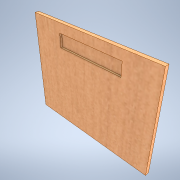
# Autodesk Inventor part: DoosjeVoorkant
Saved by Autodesk Inventor 2021 (Build 250183000, 183)
## iProperties
Created: 2021-03-11
Part Number: DoosjeVoorkant
Material: Wood (Cherry)
Document SubType Name: Modeling
Designer: ZiweZhang
Density: 0.63 g/cm^3
Appearance: Cherry - Natural Low Gloss
Author: ZiweZhang
Autodesk Inventor part; units mm, degrees
ref_plane "YZ Plane" through (0, 0, 0) normal (1, 0, 0) x (0, 1, 0)
ref_plane "XZ Plane" through (0, 0, 0) normal (0, 1, 0) x (-1, 0, 0)
ref_plane "XY Plane" through (0, 0, 0) normal (0, 0, 1) x (1, 0, 0)
sketch "Sketch1" plane through (0, 0, 0) normal (0, 0, 1) x (1, 0, 0)
  line L0 (0, 0) -> (99, 0)
  line L1 (99, 0) -> (99, 77)
  line L2 (99, 77) -> (0, 77)
  line L3 (0, 77) -> (0, 0)
  dimension "d1" = 77
  dimension "d51" = 99
  constraints: 8 end point, 2 parallel, 1 horizontal, 1 perpendicular
  measures "d1" distance of L1.end L0.end
  measures "d51" distance of L1.end L2.end
extrude "Extrusion1" add sketch "Sketch1" along normal blind 3
sketch "Sketch4" plane through (0, 0, 3) normal (0, 0, 1) x (1, 0, 0)
  line L0 (24.5, 70) -> (74.5, 70)
  line L1 (74.5, 70) -> (74.5, 60)
  line L2 (74.5, 60) -> (24.5, 60)
  line L3 (24.5, 60) -> (24.5, 70)
  line L4 (24.5, 70) -> (74.5, 60) construction
  line L5 (74.5, 70) -> (24.5, 60) construction
  line L6 (0, 77) -> (49.5, 77)
  line L7 (99, 77) -> (0, 77) projected
  point P0 (0, 0)
  dimension "d47" = 50
  dimension "d48" = 10
  constraints: 14 end point, 2 parallel, 1 horizontal, 1 midpoint, 1 perpendicular
  measures "d47" distance of L1.end L2.end
  measures "d48" distance of L0.end L1.end
extrude "Extrusion2" cut sketch "Sketch4" against normal blind 1.5
body "Solid1"
